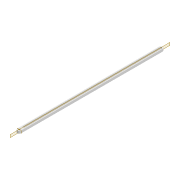
# Autodesk Inventor part: Part_6
Saved by Autodesk Inventor 2022 (Build 260153000, 153)
## iProperties
Created: 2022-04-22
Part Number: Part_6
Material: Generic
Document SubType Name: Modeling
Designer: dell
Density: 1 g/cm^3
Appearance: Default
Author: dell
Autodesk Inventor part; units mm, degrees
ref_plane "XZ Plane" through (0, 0, 0) normal (0, 1, 0) x (-1, 0, 0)
sketch "Sketch1" plane through (0, 0, 0) normal (0, 1, 0) x (-1, 0, 0)
  line L0 (0, 0) -> (0, -300) construction
  line L1 (4, 0) -> (4, -300)
  line L2 (-4, -300) -> (-4, 0)
  arc A0 (4, 0) -> (-4, 0) centre (0, 0) ccw
  arc A1 (-4, -300) -> (4, -300) centre (0, -300) ccw
  circle A2 centre (0, 0) radius 2.1
  line L3 (0, -10) -> (0, -300) construction
  line L4 (2.1, -10) -> (2.1, -300)
  line L5 (-2.1, -300) -> (-2.1, -10)
  arc A3 (2.1, -10) -> (-2.1, -10) centre (0, -10) ccw
  arc A4 (-2.1, -300) -> (2.1, -300) centre (0, -300) ccw
  point P0 (0, -150)
  point P1 (0, -155)
  dimension "d0" = 8
  dimension "d1" = 300
  dimension "d2" = 4.2
  dimension "d3" = 4.2
  dimension "d4" = 10
  constraints: 16 end point, 8 point on circle, 8 tangent, 5 centre point, 2 midpoint, 2 parallel, 1 coincident, 1 collinear, 1 point on line, 1 vertical
  measures "d0" distance between parallel lines of L2 L1
  measures "d1" distance of L0.end L0.start
  measures "d2" diameter of A2
  measures "d3" distance between parallel lines of L5 L4
  measures "d4" distance of L0.start L3.start
extrude "Extrusion1" add sketch "Sketch1" along normal blind 5
body "Solid1"
